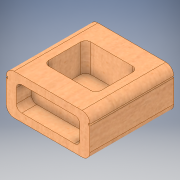
# Autodesk Inventor part: body
Saved by Autodesk Inventor 2017 (Build 210142000, 142)
## iProperties
Created: 2020-02-13
Part Number: body
Material: Wood (Cherry)
Document SubType Name: Modeling
Designer: 10023429
Density: 0.63 g/cm^3
Appearance: Cherry - Natural Low Gloss
Author: 10023429
Autodesk Inventor part; units mm, degrees
ref_plane "YZ Plane" through (0, 0, 0) normal (1, 0, 0) x (0, 1, 0)
ref_plane "XZ Plane" through (0, 0, 0) normal (0, 1, 0) x (-1, 0, 0)
ref_plane "XY Plane" through (0, 0, 0) normal (0, 0, 1) x (1, 0, 0)
sketch "Sketch1" plane through (0, 0, 0) normal (0, 0, 1) x (1, 0, 0)
  point P0 (0, 0)
sketch "Sketch2" plane through (0, 0, 0) normal (0, 0, 1) x (1, 0, 0)
  line L0 (0.3174, 0) -> (65.5954, 0)
  line L1 (73.2154, 7.62) -> (73.2154, 31.242)
  line L2 (65.5954, 38.862) -> (0.3174, 38.862)
  line L3 (-7.3026, 31.242) -> (-7.3026, 7.62)
  arc A0 (0.3174, 38.862) -> (-7.3026, 31.242) centre (0.3174, 31.242) ccw
  arc A1 (-7.3026, 7.62) -> (0.3174, 0) centre (0.3174, 7.62) ccw
  arc A2 (73.2154, 31.242) -> (65.5954, 38.862) centre (65.5954, 31.242) ccw
  arc A3 (65.5954, 0) -> (73.2154, 7.62) centre (65.5954, 7.62) ccw
  point P0 (0, 0)
  point P1 (-7.3026, 0)
  point P2 (73.2154, 0)
  point P3 (73.2154, 38.862)
  dimension "d0" = 80.518
  dimension "d1" = 38.862
  dimension "d2" = 7.62
  constraints: 8 end point, 8 point on circle, 8 tangent, 6 point on line, 4 centre point, 3 equal radius, 2 horizontal, 2 perpendicular
  measures "d0" distance of point (-7.303, 0) point (73.215, 0)
  measures "d1" distance of point (73.215, 0) point (73.215, 38.862)
  measures "d2" radius of A0
extrude "Extrusion1" add sketch "Sketch2" along normal blind 80.518
sketch "Sketch3" plane through (0, 0, 80.518) normal (0, 0, 1) x (1, 0, 0)
  line L0 (7.5564, 7.62) -> (58.3564, 7.62)
  line L1 (63.4364, 12.7) -> (63.4364, 26.162)
  line L2 (58.3564, 31.242) -> (7.5564, 31.242)
  line L3 (2.4764, 26.162) -> (2.4764, 12.7)
  line L4 (73.2154, 7.62) -> (73.2154, 31.242) projected
  line L5 (65.5954, 38.862) -> (0.3174, 38.862) projected
  arc A0 (7.5564, 31.242) -> (2.4764, 26.162) centre (7.5564, 26.162) ccw
  arc A1 (2.4764, 12.7) -> (7.5564, 7.62) centre (7.5564, 12.7) ccw
  arc A2 (58.3564, 7.62) -> (63.4364, 12.7) centre (58.3564, 12.7) ccw
  arc A3 (63.4364, 26.162) -> (58.3564, 31.242) centre (58.3564, 26.162) ccw
  point P0 (0, 0)
  point P1 (2.4764, 7.62)
  point P2 (63.4364, 7.62)
  point P3 (63.4364, 31.242)
  dimension "d5" = 60.96
  dimension "d6" = 23.622
  dimension "d7" = 9.779
  dimension "d8" = 7.62
  dimension "d9" = 5.08
  constraints: 8 end point, 8 point on circle, 8 tangent, 6 point on line, 4 centre point, 3 equal radius, 2 horizontal, 2 perpendicular
  measures "d5" distance of point (2.476, 7.62) point (63.436, 7.62)
  measures "d6" distance of point (63.436, 7.62) point (63.436, 31.242)
  measures "d7" distance between parallel lines of L4 L1
  measures "d8" distance between parallel lines of L5 L2
  measures "d9" radius of A0
extrude "Extrusion2" cut sketch "Sketch3" against normal blind 14.478
sketch "Sketch4" plane through (0.3174, 38.862, 0) normal (0, 1, 0) x (1, 0, 0)
  line L0 (12.573, -19.304) -> (52.705, -19.304)
  line L1 (57.785, -24.384) -> (57.785, -54.61)
  line L2 (52.705, -59.69) -> (12.573, -59.69)
  line L3 (7.493, -54.61) -> (7.493, -24.384)
  line L4 (65.278, -80.518) -> (0, -80.518) projected
  line L5 (72.898, 0) -> (72.898, -80.518) projected
  arc A0 (7.493, -54.61) -> (12.573, -59.69) centre (12.573, -54.61) ccw
  arc A1 (12.573, -19.304) -> (7.493, -24.384) centre (12.573, -24.384) ccw
  arc A2 (57.785, -24.384) -> (52.705, -19.304) centre (52.705, -24.384) ccw
  arc A3 (52.705, -59.69) -> (57.785, -54.61) centre (52.705, -54.61) ccw
  point P0 (-0.3174, 0)
  point P1 (7.493, -19.304)
  point P2 (57.785, -19.304)
  point P3 (57.785, -59.69)
  point P4 (7.493, -59.69)
  dimension "d12" = 50.292
  dimension "d13" = 40.386
  dimension "d14" = 20.828
  dimension "d15" = 15.113
  dimension "d18" = 5.08
  constraints: 8 end point, 8 point on circle, 8 point on line, 8 tangent, 4 centre point, 3 equal radius, 2 perpendicular, 1 horizontal, 1 vertical
  measures "d12" distance of point (7.493, -19.304) point (57.785, -19.304)
  measures "d13" distance of point (57.785, -19.304) point (57.785, -59.69)
  measures "d14" distance between parallel lines of L4 L2
  measures "d15" distance between parallel lines of L1 L5
  measures "d18" radius of A0
extrude "Extrusion3" cut sketch "Sketch4" against normal blind 27.178
sketch "Sketch5" plane through (0, 0, 80.518) normal (0, 0, 1) x (1, 0, 0)
  line L0 (73.2154, 7.62) -> (73.2154, 31.242) projected
  line L1 (73.2154, 31.242) -> (71.6914, 31.242)
  line L2 (71.6914, 31.242) -> (71.6914, 29.718)
  line L3 (71.6914, 29.718) -> (73.2154, 29.718)
  line L4 (73.2154, 31.242) -> (73.2154, 29.718)
  line L5 (65.5954, 38.862) -> (0.3174, 38.862) projected
  point P0 (0, 0)
  dimension "d19" = 1.524
  dimension "d20" = 1.524
  dimension "d21" = 7.62
  constraints: 8 end point, 2 perpendicular, 1 horizontal, 1 vertical
  measures "d19" distance of L0.end L1.end
  measures "d20" distance of L1.end L2.end
  measures "d21" distance between parallel lines of L1 L5
extrude "Extrusion4" cut sketch "Sketch5" against normal blind 80.518
sketch "Sketch6" plane through (0, 0, 80.518) normal (0, 0, 1) x (1, 0, 0)
  line L0 (-7.3026, 31.242) -> (-7.3026, 7.62) projected
  line L1 (-7.3026, 31.242) -> (-5.7786, 31.242)
  line L2 (-5.7786, 31.242) -> (-5.7786, 29.718)
  line L3 (-5.7786, 29.718) -> (-7.3026, 29.718)
  line L4 (-7.3026, 31.242) -> (-7.3026, 29.718)
  point P0 (0, 0)
  dimension "d24" = 1.524
  dimension "d25" = 1.524
  constraints: 8 end point, 3 perpendicular, 1 horizontal, 1 point on line
  measures "d24" distance of L0.start L1.end
  measures "d25" distance of L1.end L2.end
extrude "Extrusion5" cut sketch "Sketch6" against normal blind 80.518
body "Solid1"
